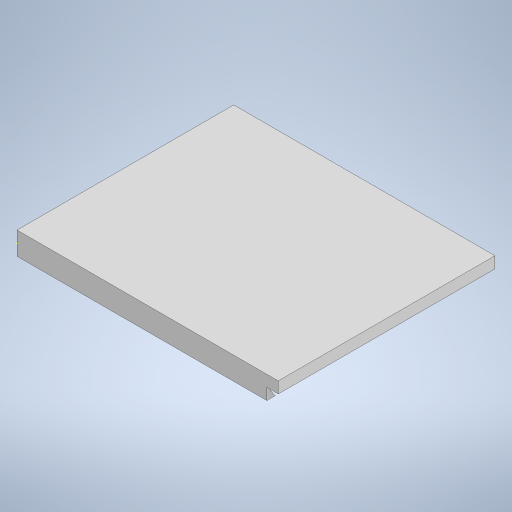
# Autodesk Inventor part: tapa_pcb
Saved by Autodesk Inventor 2024.3 (Build 283343000, 343)
## iProperties
Created: 2025-07-17
Part Number: tapa_pcb
Material: Genérico
Document SubType Name: Modeling
Designer: Damian
Density: 1 g/cm^3
Appearance: Valor por defecto
Author: Damian
Autodesk Inventor part; units mm, degrees
ref_plane "YZ Plane" through (0, 0, 0) normal (1, 0, 0) x (0, 1, 0)
ref_plane "XZ Plane" through (0, 0, 0) normal (0, 1, 0) x (-1, 0, 0)
ref_plane "XY Plane" through (0, 0, 0) normal (0, 0, 1) x (1, 0, 0)
sketch "Boceto1" plane through (0, 0, 0) normal (1, 0, 0) x (0, 1, 0)
  point P0 (0, 0)
sketch "Boceto2" plane through (0, 0, 0) normal (1, 0, 0) x (0, 1, 0)
  line L0 (0, 0) -> (0, -95.4)
  line L1 (0, -95.4) -> (5, -95.4)
  line L2 (5, -95.4) -> (5, 0)
  line L3 (5, 0) -> (0, 0)
  line L4 (0, 0) -> (-5, 0)
  line L5 (-5, 0) -> (-5, -3.75)
  line L6 (-5, -3.75) -> (-2.25, -1.75)
  line L7 (-2.25, -1.75) -> (0, -1.75)
  line L8 (11.8488, -47.7) -> (-15.1149, -47.7) construction
  line L9 (0, -95.4) -> (-5, -95.4)
  line L10 (-5, -95.4) -> (-5, -91.65)
  line L11 (-5, -91.65) -> (-2.25, -93.65)
  line L12 (-2.25, -93.65) -> (0, -93.65)
  point P0 (-1.125, -1.75)
  point P1 (5, -47.7)
  point P2 (0, -93.65)
  dimension "d0" = 5
  dimension "d1" = 95.4
  dimension "d2" = 5
  dimension "d4" = 3.75
  dimension "d5" = 1.75
  dimension "d6" = 2.25
  dimension "d7" = 0
  constraints: 26 end point, 4 perpendicular, 4 symmetric about line, 2 horizontal, 2 midpoint, 1 parallel, 1 point on line, 1 vertical
  measures "d0" distance of L0.end L1.end
  measures "d1" distance of L1.end L2.end
  measures "d2" distance of L0.start L4.end
  measures "d4" distance of L4.end L5.end
  measures "d5" distance from line of point (-1.125, -1.75) L4
  measures "d6" distance of L6.end L7.end
  measures "d7" distance from line of point (5, -47.7) L8
extrude "Extrusión1" add sketch "Boceto2" along normal blind 110 contours L0 L7 L6 L5 L4 | L0 L9 L10 L11 L12
extrude "Extrusión2" add sketch "Boceto2" along normal blind 115 contours L3 L2 L1 L0
